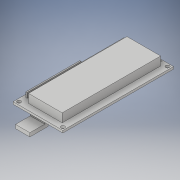
# Autodesk Inventor part: LCD_Screen
Saved by Autodesk Inventor 2018 (Build 220112000, 112)
## iProperties
Created: 2020-03-26
Part Number: LCD_Screen
Material: Generic
Document SubType Name: Modeling
Designer: natha
Density: 1 g/cm^3
Appearance: Default
Author: natha
Autodesk Inventor part; units mm, degrees
ref_plane "YZ Plane" through (0, 0, 0) normal (1, 0, 0) x (0, 1, 0)
ref_plane "XZ Plane" through (0, 0, 0) normal (0, 1, 0) x (-1, 0, 0)
ref_plane "XY Plane" through (0, 0, 0) normal (0, 0, 1) x (1, 0, 0)
sketch "Sketch1" plane through (0, 0, 0) normal (0, 1, 0) x (-1, 0, 0)
  line L0 (0, 0) -> (36, 0)
  line L1 (36, 0) -> (36, -80)
  line L2 (36, -80) -> (0, -80)
  line L3 (0, -80) -> (0, 0)
  circle A0 centre (33.85, -77.85) radius 1.35
  circle A1 centre (2.15, -77.85) radius 1.35
  circle A2 centre (33.85, -2.15) radius 1.35
  circle A3 centre (2.15, -2.15) radius 1.35
  dimension "d0" = 36
  dimension "d1" = 80
  dimension "d2" = 2.7
  dimension "d3" = 2.15
  dimension "d4" = 2.15
  dimension "d5" = 2.7
  dimension "d6" = 2.15
  dimension "d7" = 2.7
  dimension "d8" = 2.15
  dimension "d9" = 2.7
  constraints: 8 end point, 4 centre point, 2 parallel, 1 horizontal, 1 perpendicular
  measures "d0" distance of L1.end L2.end
  measures "d1" distance of L0.end L1.end
  measures "d2" diameter of A0
  measures "d3" distance from line of L2 A0.centre
  measures "d4" distance from line of L1 A0.centre
  measures "d5" diameter of A1
  measures "d6" distance from line of L3 A1.centre
  measures "d7" diameter of A2
  measures "d8" distance from line of L0 A2.centre
  measures "d9" diameter of A3
extrude "Extrusion1" add sketch "Sketch1" along normal blind 1.6
sketch "Sketch2" plane through (0, 1.6, 0) normal (0, 1, 0) x (1, 0, 0)
  line L0 (-29.35, 4.5) -> (-5, 4.5)
  line L1 (-5, 4.5) -> (-5, 75.7)
  line L2 (-5, 75.7) -> (-29.35, 75.7)
  line L3 (-29.35, 75.7) -> (-29.35, 4.5)
  line L4 (-36, 0) -> (0, 0) projected
  line L5 (0, 0) -> (0, 80) projected
  dimension "d12" = 24.35
  dimension "d13" = 71.2
  dimension "d14" = 4.5
  dimension "d15" = 5
  constraints: 8 end point, 2 parallel, 1 horizontal, 1 perpendicular
  measures "d12" distance of L2.end L1.end
  measures "d13" distance of L1.end L0.end
  measures "d14" distance between parallel lines of L0 L4
  measures "d15" distance between parallel lines of L1 L5
extrude "Extrusion2" add sketch "Sketch2" along normal blind 6.25
sketch "Sketch3" plane through (0, 1.6, 0) normal (0, 1, 0) x (1, 0, 0)
  line L0 (-34, 7.1651) -> (-33, 7.1651)
  line L1 (-33, 7.1651) -> (-33, 46.1651)
  line L2 (-33, 46.1651) -> (-34, 46.1651)
  line L3 (-34, 46.1651) -> (-34, 7.1651)
  line L4 (-36, 80) -> (-36, 0) projected
  point P0 (0, 0)
  dimension "d18" = 1
  dimension "d19" = 39
  dimension "d20" = 2
  constraints: 8 end point, 2 parallel, 1 horizontal, 1 perpendicular
  measures "d18" distance of L2.end L1.end
  measures "d19" distance of L1.end L0.end
  measures "d20" distance between parallel lines of L4 L3
extrude "Extrusion3" add sketch "Sketch3" along normal blind 3.6
sketch "Sketch4" plane through (-5, 1.6, -75.7) normal (0, 0, -1) x (-1, 0, 0)
  line L0 (-5, 0) -> (31, 0) projected
  line L1 (2.5, 0) -> (21.85, 0)
  line L2 (21.85, 0) -> (21.85, 2.3329)
  line L3 (21.85, 2.3329) -> (2.5, 2.3329)
  line L4 (2.5, 2.3329) -> (2.5, 0)
  line L5 (0, 0) -> (0, 6.25) projected
  line L6 (24.35, 0) -> (24.35, 6.25) projected
  point P0 (-5, -1.6)
  dimension "d23" = 2.5
  dimension "d24" = 2.5
  constraints: 8 end point, 2 parallel, 1 horizontal, 1 perpendicular, 1 point on line
  measures "d23" distance between parallel lines of L4 L5
  measures "d24" distance between parallel lines of L6 L2
extrude "Extrusion4" add sketch "Sketch4" along normal blind 3.6
sketch "Sketch5" plane through (-26.85, 3.9329, -75.7) normal (0, 1, 0) x (1, 0, 0)
  line L0 (19.35, 0) -> (15.75, 3.6)
  line L1 (19.35, 0) -> (24.4412, 0) construction
  line L2 (0, 0) -> (3.6, 3.6)
  line L3 (0, 0) -> (5.0912, 0) construction
  line L4 (3.6, 3.6) -> (15.75, 3.6)
  line L5 (19.35, 3.6) -> (19.35, 0) projected
  line L6 (19.35, 0) -> (19.35, 3.6)
  line L7 (19.35, 3.6) -> (15.75, 3.6)
  line L8 (3.6, 3.6) -> (0, 3.6)
  line L9 (0, 0) -> (0, 3.6)
  line L10 (21.85, 0) -> (-2.5, 0) projected
  point P0 (26.85, -75.7)
  dimension "d27" = 135
  dimension "d28" = 45
  constraints: 18 end point, 2 equal length, 2 horizontal, 2 perpendicular, 1 vertical
  measures "d27" angle of L1 L0
  measures "d28" angle of L3 L2
extrude "Extrusion5" cut sketch "Sketch5" against normal blind 2.333 contours L0 L7 L5 | L9 L8 L2
sketch "Sketch6" plane through (0, 0, 0) normal (0, -1, 0) x (1, 0, 0)
  line L0 (-34.5, -6) -> (-15.15, -6)
  line L1 (-15.15, -6) -> (-15.15, -48)
  line L2 (-15.15, -48) -> (-34.5, -48)
  line L3 (-34.5, -48) -> (-34.5, -6)
  line L4 (-36, 0) -> (-36, -80) projected
  line L5 (0, 0) -> (-36, 0) projected
  dimension "d31" = 19.35
  dimension "d32" = 42
  dimension "d33" = 1.5
  dimension "d34" = 6
  constraints: 8 end point, 2 parallel, 1 horizontal, 1 perpendicular
  measures "d31" distance of L1.end L2.end
  measures "d32" distance of L0.end L1.end
  measures "d33" distance between parallel lines of L4 L3
  measures "d34" distance between parallel lines of L5 L0
extrude "Extrusion6" add sketch "Sketch6" along normal blind 4.15
sketch "Sketch7" plane through (0, -4.15, 0) normal (0, -1, 0) x (1, 0, 0)
  line L0 (-15.15, -6) -> (-34.5, -6) projected
  line L1 (-29.5, -6) -> (-19.1, -6)
  line L2 (-19.1, -6) -> (-19.1, -8.4)
  line L3 (-19.1, -8.4) -> (-29.5, -8.4)
  line L4 (-29.5, -8.4) -> (-29.5, -6)
  line L5 (-34.5, -6) -> (-34.5, -48) projected
  point P0 (0, 0)
  dimension "d37" = 10.4
  dimension "d38" = 2.4
  dimension "d39" = 5
  constraints: 8 end point, 2 parallel, 1 horizontal, 1 perpendicular, 1 point on line
  measures "d37" distance of L2.end L3.end
  measures "d38" distance of L1.end L2.end
  measures "d39" distance between parallel lines of L4 L5
extrude "Extrusion7" add sketch "Sketch7" along normal blind 5.5
sketch "Sketch8" plane through (-34.5, 0, -6) normal (0, 0, 1) x (1, 0, 0)
  line L0 (15.4, -9.65) -> (5, -9.65) projected
  line L1 (15.4, -4.15) -> (15.4, -9.65) projected
  line L2 (5, -9.65) -> (15.4, -9.65)
  line L3 (15.4, -9.65) -> (15.4, -7)
  line L4 (15.4, -7) -> (5, -7)
  line L5 (5, -7) -> (5, -9.65)
  point P0 (34.5, 0)
  dimension "d42" = 2.65
  constraints: 8 end point, 2 parallel, 1 horizontal, 1 perpendicular, 1 point on line
  measures "d42" distance of L3.end L2.end
extrude "Extrusion8" add sketch "Sketch8" along normal blind 10.75
body "Solid1"
